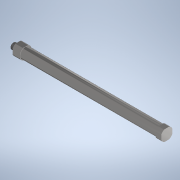
# Autodesk Inventor part: CJ2B16-200Z(1_0)_BODY
Saved by Autodesk Inventor 2020.2 (Build 242310000, 310)
## iProperties
Created: 2020-03-06
Part Number: CJ2B16-200Z(1_0)_BODY
Material: 鉄、鋳鉄
Catalog Web Link: www.cadenas.de
Description: CJ2-Z BODY-Air Cylinder/Standard: Double Acting Single Rod
Vendor: SMC
Document SubType Name: Modeling
Designer: psadmin
Manufacturer: SMC
Mass: 134.868 g
Surface Area: 257.248 cm^2
Volume: 18.8626 cm^3
Density: 7.15 g/cm^3
Appearance: 鋼 - つや出し
Category: PARTsolutions
Company: SMC
PSOL_IDENT_0: {$CADENAS_DATA\23d-libs\smc_jp\actuator\standard_air_cylinder\cj2\cj2_z\parts\cj2_z_body.prj},263 {V
PSOL_IDENT_1: TYP=3D},{NB=CJ2B16-200Z(1_0)_BODY},{LINA=CJ2B16-200Z_BODY},{NN=CJ2-Z BODY},{DATE=06.02.2020 05:07:19
PSOL_IDENT_2: },{GEOMDATE=19.11.2018 05:34:00},{VERSION=},{LINEID=410},{WBVAR=AUTOSWITCH,NUMBER,CUSHION,STOP,STROK
PSOL_IDENT_3: E,PORT,MOUNTING,OMSCXC3,OMSCXC51,THREAD},{WBNUMERIC=STROKE}  {NB=CJ2B16-200Z(1_0)_BODY},{LINA=CJ2B16
PSOL_IDENT_4: -200Z_BODY},{KT=DUMMY},{ORDER=CJ2B16-200Z},{BORE=16},{MOUNT=(B) Basic},{AUTOSWITCH=},{NUMBER=},{CUSH
PSOL_IDENT_5: ION=},{MOUNTX=B},{STOP=1},{STROKE=200},{SMAX=400},{PORT=},{MOUNTING=},{OMSCXC3=},{OMSCXC51=},{THREAD=
PSOL_IDENT_6: 0},{B=18.3},{B1X1=18.3},{B2=18.300},{C=20},{C1X1=20.0},{C2=20.000},{CD=0.0},{U=0},{CX=0.0},{CZ=0},{C
PSOL_IDENT_7: Z1X1=0.0},{D=5},{F=8},{GA=8.0},{GA1X1=8.0},{GA2=7.500},{GB=5.0},{GB1X1=5.0},{GB2=6.500},{H=28},{NA=1
PSOL_IDENT_8: 2.5},{NA1X1=12.5},{NA2=21.000},{NB1=9.5},{NB1X1=9.5},{NB2=20.000},{NDH8=10 0/-0.022},{NDH81=10},{NN=
PSOL_IDENT_9: M10x1.0},{NN1=10},{NN2=1.0},{R=0},{S=47},{S1X1=47.0},{S2X2=66.000},{WA=14.5},{WB=13.5},{WW=5.5},{MOU
PSOL_IDENT_10: NTINGX='','(-) None','-A','(A) Rail mounting','-B','(B) Band mounting'},{PORTX='', '(-) Perpendicula
PSOL_IDENT_11: r', 'R', '(R) In-line'},{SWX=5},{SW1=6.500},{SW2=2.500},{SW3=3.000},{SW4=2.000},{SW5=5.000},{SW6=1.0
PSOL_IDENT_12: 00},{SW7=3.500},{SW8=4.000},{SW9=1.000},{SW=5},{SWSINX= '','N/A' },{NENN=CJ2B16},{X1=6.000},{X2=7.50
PSOL_IDENT_13: 0},{Y1=3.000},{Y2=6.500},{X=6},{Y=3},{XC3= '','(-) None','-XC3AB','(XC3AB) Rod port location viewed:
PSOL_IDENT_14: A,Head port location viewed: B','-XC3AC','(XC3AC) Rod port location viewed: A,Head port location vi
PSOL_IDENT_15: ewed: C','-XC3AD','(XC3AD) Rod port location viewed: A,Head port location viewed: D','-XC3BA','(XC3B
PSOL_IDENT_16: A) Rod port location viewed: B,Head port location viewed: A','-XC3BB','(XC3BB) Rod port location vie
PSOL_IDENT_17: wed: B,Head port location viewed: B','-XC3BC','(XC3BC) Rod port location viewed: B,Head port locatio
PSOL_IDENT_18: n viewed: C','-XC3BD','(XC3BD) Rod port location viewed: B,Head port location viewed:D','-XC3CA','(X
PSOL_IDENT_19: C3CA) Rod port location viewed: C,Head port location viewed: A','-XC3CB','(XC3CB) Rod port location
PSOL_IDENT_20: viewed: C,Head port location viewed: B','-XC3CC','(XC3CC) Rod port location viewed: C,Head port loca
PSOL_IDENT_21: tion viewed: C','-XC3CD','(XC3CD) Rod port location viewed: C,Head port location viewed:D','-XC3DA','
PSOL_IDENT_22: (XC3DA) Rod port location viewed: D,Head port location viewed: A','-XC3DB','(XC3DB) Rod port locatio
PSOL_IDENT_23: n viewed: D,Head port location viewed: B','-XC3DC','(XC3DC) Rod port location viewed: D,Head port lo
PSOL_IDENT_24: cation viewed: C','-XC3DD','(XC3DD) Rod port location viewed: D,Head port location viewed:D' },{PORT
PSOL_IDENT_25: XC3=A1},{PORTXC32=A2},{CUSHIONX= '','(-) Rubber cushion','A','(A) Air cushion' },{XC51= '','(-) None'
PSOL_IDENT_26: ,'-XC51H4','(XC51H4) Hose nipple type: ø4/2.5 with restriction','-XC51H6','(XC51H6) Hose nipple type
PSOL_IDENT_27: : ø6/4 with restriction','-XC51MH4','(XC51MH4) Hose nipple type: ø4/2.5 without restriction','-XC51M
PSOL_IDENT_28: H6','(XC51MH6) Hose nipple type: ø6/4 without restriction' },{MODEL=M-5H-6},{PINMODEL=CD-Z015}
NN: M10x1.0
NT: Air Cylinder/Standard: Double Acting Single Rod
NB: CJ2B16-200Z(1_0)_BODY
NBSYN: $ORDER.($STOP._$THREAD.)_BODY
LINA: CJ2B16-200Z_BODY
ROWDESC: CJ2B16
BORE: 16
MOUNT: (B) Basic
AUTOSWITCH: (-) Without autoswitch
NUMBER: N/A
CUSHION: (-) Rubber cushion
STOP: Manufacturable stroke
STROKE: 200
SMAX: 400
PORT: (-) Perpendicular
MOUNTING: (-) None
OMSCXC3: (-) None
OMSCXC51: (-) None
THREAD: on
B: 18.3
B1X1: 18.3
B2: 18.3
C: 20
C1X1: 20
C2: 20
CD: 0
U: 0
CX: 0
CZ: 0
CZ1X1: 0
D: 5
F: 8
GA: 8
GA1X1: 8
GA2: 7.5
GB: 5
GB1X1: 5
GB2: 6.5
H: 28
NA: 12.5
NA1X1: 12.5
NA2: 21
NB1: 9.5
NB1X1: 9.5
NB2: 20
NDH8: 10 0/-0.022
NDH81: 10
NN1: 10
NN2: 1
R: 0
S: 47
S1X1: 47
S2X2: 66
WA: 14.5
WB: 13.5
WW: 5.5
SW1: 6.5
SW2: 2.5
SW3: 3
SW4: 2
SW5: 5
SW6: 1
SW7: 3.5
SW8: 4
SW9: 1
X1: 6
X2: 7.5
Y1: 3
Y2: 6.5
SUPPLIER: SMC
ARTICLENO: CJ2B16-200Z(1_0)_BODY
BOMINFO: CJ2B16-200Z_BODY
CREATOR: CADENAS GmbH
Title: CJ2B16-200Z_BODY
Author: Cadenas PARTsolutions
Comments: Air Cylinder/Standard: Double Acting Single Rod
Autodesk Inventor part; units mm, degrees
sketch "Sketch_8" plane through (0, 0, 0) normal (0, 0, 1) x (1, 0, 0)
  line L0 (0, 0) -> (-8, 0)
  line L1 (-8, 0) -> (-8, 4.3865)
  line L2 (-8, 4.3865) -> (-7.3865, 5)
  line L3 (-7.3865, 5) -> (0, 5)
  line L4 (0, 5) -> (0, 0)
  line L5 (0, 0) -> (-8, 0)
  constraints: 12 end point
revolve "Revolution1" add sketch "Sketch_8" angle 360 about axis through (0, 0, 0) along (1, 0, 0)
thread "Thread1" size "M10x1" class "6g" standard "ISO Metric profile" length 5.8865
sketch "Sketch_9" plane through (0, 0, 0) normal (1, 0, 0) x (0, 0, -1)
  line L0 (-9.15, 4.0345) -> (-9.15, -4.0345)
  arc A0 (-9.15, -4.0345) -> (-4.0345, -9.15) centre (0, 0) ccw
  line L1 (-4.0345, -9.15) -> (4.0345, -9.15)
  arc A1 (4.0345, -9.15) -> (9.15, -4.0345) centre (0, 0) ccw
  line L2 (9.15, -4.0345) -> (9.15, 4.0345)
  arc A2 (9.15, 4.0345) -> (4.0345, 9.15) centre (0, 0) ccw
  line L3 (4.0345, 9.15) -> (-4.0345, 9.15)
  arc A3 (-4.0345, 9.15) -> (-9.15, 4.0345) centre (0, 0) ccw
  constraints: 8 end point, 8 point on circle, 4 centre point
extrude "Extrusion1" add sketch "Sketch_9" along normal blind 12.5
sketch "Sketch_11" plane through (12.5, 0, 0) normal (1, 0, 0) x (0, 0, -1)
  circle A0 centre (0, 0) radius 8.7
  constraints: 1 centre point
extrude "Extrusion2" add sketch "Sketch_11" along normal blind 225
sketch "Sketch_10" plane through (237.5, 0, 0) normal (1, 0, 0) x (0, 0, -1)
  line L0 (-9.15, 4.0345) -> (-9.15, -4.0345)
  arc A0 (-9.15, -4.0345) -> (-4.0345, -9.15) centre (0, 0) ccw
  line L1 (-4.0345, -9.15) -> (4.0345, -9.15)
  arc A1 (4.0345, -9.15) -> (9.15, -4.0345) centre (0, 0) ccw
  line L2 (9.15, -4.0345) -> (9.15, 4.0345)
  arc A2 (9.15, 4.0345) -> (4.0345, 9.15) centre (0, 0) ccw
  line L3 (4.0345, 9.15) -> (-4.0345, 9.15)
  arc A3 (-4.0345, 9.15) -> (-9.15, 4.0345) centre (0, 0) ccw
  constraints: 8 end point, 8 point on circle, 4 centre point
extrude "Extrusion3" add sketch "Sketch_10" along normal blind 9.5
sketch "Sketch7" plane through (0, 0, 0) normal (0, 0, 1) x (1, 0, 0)
  line L0 (8, 9.15) -> (8, 4.15)
  line L1 (8, 2.9566) -> (5.933, 4.15)
  line L2 (5.933, 4.15) -> (5.933, 8.717)
  line L3 (5.933, 8.717) -> (5.5, 9.15)
  line L4 (5.5, 9.15) -> (8, 9.15)
  line L5 (8, 9.15) -> (8, 2.9566)
  constraints: 12 end point
revolve "Revolution2" cut sketch "Sketch7" angle 360 about axis through (8, 9.15, 0) along (0, 1, 0)
thread "Thread2" size "M5x0.8" class "6H" standard "ISO Metric profile" full length
sketch "Sketch_7" plane through (0, 0, 0) normal (0, 0, 1) x (1, 0, 0)
  line L0 (242, 9.15) -> (242, 4.15)
  line L1 (242, 2.9566) -> (239.933, 4.15)
  line L2 (239.933, 4.15) -> (239.933, 8.717)
  line L3 (239.933, 8.717) -> (239.5, 9.15)
  line L4 (239.5, 9.15) -> (242, 9.15)
  line L5 (242, 9.15) -> (242, 2.9566)
  constraints: 12 end point
revolve "Revolution3" cut sketch "Sketch_7" angle 360 about axis through (242, 9.15, 0) along (0, 1, 0)
thread "Thread3" size "M5x0.8" class "6H" standard "ISO Metric profile" full length
sketch "Sketch_16" plane through (0, 0, 0) normal (0, 0, 1) x (1, 0, 0)
  line L0 (217.5, 0) -> (-8, 0)
  line L1 (-8, 0) -> (-8, 2.5)
  line L2 (-8, 2.5) -> (12.5, 2.5)
  line L3 (12.5, 2.5) -> (12.5, 8)
  line L4 (12.5, 8) -> (217.5, 8)
  line L5 (217.5, 8) -> (217.5, 0)
  line L6 (217.5, 0) -> (-8, 0)
  constraints: 14 end point
revolve "Revolution4" cut sketch "Sketch_16" angle 360 about axis through (217.5, 0, 0) along (1, 0, 0)
ref_plane "BODY_N_XY" through (247, 0, 0) normal (0, 0, -1) x (1, 0, 0)
ref_plane "BODY_N_YZ" through (247, 0, 0) normal (1, 0, 0) x (0, -1, 0)
ref_plane "BODY_N_ZX" through (247, 0, 0) normal (0, -1, 0) x (0, 0, -1)
ref_plane "NUT2_XY" through (247, 0, 0) normal (1, 0, 0) x (0, 0, -1)
ref_plane "NUT2_YZ" through (247, 0, 0) normal (0, 0, -1) x (0, 1, 0)
ref_plane "NUT2_ZX" through (247, 0, 0) normal (0, 1, 0) x (1, 0, 0)
ref_plane "SW1_XY" through (17.5, 0, 0) normal (1, 0, 0) x (0, 0, -1)
ref_plane "SW1_YZ" through (17.5, 0, 0) normal (0, 0, -1) x (0, 1, 0)
ref_plane "SW1_ZX" through (17.5, 0, 0) normal (0, 1, 0) x (1, 0, 0)
ref_plane "SW2_XY" through (232.5, 0, 0) normal (-1, 0, 0) x (0, 0, -1)
ref_plane "SW2_YZ" through (232.5, 0, 0) normal (0, 0, -1) x (0, -1, 0)
ref_plane "SW2_ZX" through (232.5, 0, 0) normal (0, -1, 0) x (-1, 0, 0)
ref_plane "SW_R1_XY" through (17.5, -14.15, 0) normal (1, 0, 0) x (0, 0, -1)
ref_plane "SW_R1_YZ" through (17.5, -14.15, 0) normal (0, 0, -1) x (0, 1, 0)
ref_plane "SW_R1_ZX" through (17.5, -14.15, 0) normal (0, 1, 0) x (1, 0, 0)
ref_plane "SW_R2_XY" through (232.5, -14.15, 0) normal (-1, 0, 0) x (0, 0, -1)
ref_plane "SW_R2_YZ" through (232.5, -14.15, 0) normal (0, 0, -1) x (0, -1, 0)
ref_plane "SW_R2_ZX" through (232.5, -14.15, 0) normal (0, -1, 0) x (-1, 0, 0)
ref_plane "body_XY" through (0, 0, 0) normal (1, 0, 0) x (0, 0, -1)
ref_plane "body_YZ" through (0, 0, 0) normal (0, 0, -1) x (0, 1, 0)
ref_plane "body_ZX" through (0, 0, 0) normal (0, 1, 0) x (1, 0, 0)
body "Solid1"
